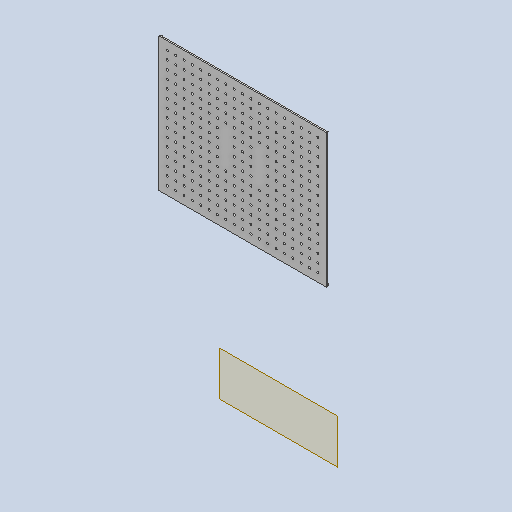
# Autodesk Inventor part: attachments_hub
Saved by Autodesk Inventor 2024.3 (Build 283343000, 343)
## iProperties
Created: 2026-05-03
Part Number: attachments_hub
Material: Generic
Document SubType Name: Modeling
Designer: owozn
Density: 1 g/cm^3
Appearance: Default
Author: owozn
Autodesk Inventor part; units mm, degrees
ref_plane "YZ Plane" through (0, 0, 0) normal (1, 0, 0) x (0, 1, 0)
ref_plane "XZ Plane" through (0, 0, 0) normal (0, 1, 0) x (-1, 0, 0)
ref_plane "XY Plane" through (0, 0, 0) normal (0, 0, 1) x (1, 0, 0)
ref_plane "Work Plane1" through (13.6818, -331.3189, 0) normal (0, 0, 1) x (1, 0, 0)
sketch "Sketch1" plane through (13.6818, -331.3189, 0) normal (0, 0, 1) x (1, 0, 0)
  line L0 (-13.6818, 214.2062) -> (-13.6818, 284.2062) projected
  line L1 (-49.9333, 331.3189) -> (45.2667, 331.3189) projected
  line L2 (-47.6818, 361.3189) -> (-37.6818, 361.3189)
  line L3 (-37.6818, 361.3189) -> (-37.6818, 311.3189)
  line L4 (-37.6818, 311.3189) -> (-47.6818, 311.3189)
  line L5 (-47.6818, 311.3189) -> (-47.6818, 361.3189)
  line L6 (-47.6818, 361.3189) -> (-37.6818, 311.3189) construction
  line L7 (-37.6818, 361.3189) -> (-47.6818, 311.3189) construction
  line L8 (20.3182, 361.3189) -> (10.3182, 361.3189)
  line L9 (10.3182, 361.3189) -> (10.3182, 311.3189)
  line L10 (10.3182, 311.3189) -> (20.3182, 311.3189)
  line L11 (20.3182, 311.3189) -> (20.3182, 361.3189)
  line L12 (20.3182, 361.3189) -> (10.3182, 311.3189) construction
  line L13 (10.3182, 361.3189) -> (20.3182, 311.3189) construction
  point P0 (-13.6818, 331.3189)
  point P1 (-42.6818, 336.3189)
  point P2 (15.3182, 336.3189)
  dimension "d0" = 10
  dimension "d1" = 50
  dimension "d2" = 29
  dimension "d3" = 5
  constraints: 24 end point, 5 symmetric about line, 2 midpoint, 2 parallel, 1 horizontal, 1 perpendicular
  measures "d0" distance of L3.end L4.end
  measures "d1" distance of L2.end L3.end
  measures "d2" distance from line of L0 point (-42.682, 336.319)
  measures "d3" distance from line of L1 point (-42.682, 336.319)
extrude "Extrusion1" add sketch "Sketch1" along normal blind 35
sketch "Sketch2" plane through (24, -20, 0) normal (-1, 0, 0) x (0, 0, 1)
  line L0 (0, -10) -> (0, 60) projected
  line L1 (-7, 20) -> (42, 20) projected
  circle A0 centre (7, 25) radius 1.6
  circle A1 centre (7, 41) radius 1.6
  line L2 (8.6, 25) -> (8.6, 41)
  line L3 (5.4, 25) -> (5.4, 41)
  point P0 (0, 20)
  dimension "d6" = 3.2
  dimension "d7" = 3.2
  dimension "d8" = 7
  dimension "d9" = 7
  dimension "d10" = 21
  dimension "d11" = 5
  constraints: 4 end point, 4 point on circle, 4 tangent, 2 centre point
  measures "d6" diameter of A0
  measures "d7" diameter of A1
  measures "d8" distance from line of L0 A0.centre
  measures "d9" distance from line of L0 A1.centre
  measures "d10" distance from line of L1 A1.centre
  measures "d11" distance from line of L1 A0.centre
extrude "Extrusion2" cut sketch "Sketch2" along normal through all both and the other way through all
sketch "Sketch3" plane through (13.6818, -331.3189, 35) normal (0, 0, 1) x (1, 0, 0)
  line L0 (-13.6818, 100.7837) -> (-13.6818, 404.7415) projected
  line L1 (-177.3333, 331.3189) -> (172.6667, 331.3189) projected
  line L2 (111.3182, 231.3189) -> (-138.6818, 231.3189)
  line L3 (-138.6818, 231.3189) -> (-138.6818, 431.3189)
  line L4 (-138.6818, 431.3189) -> (111.3182, 431.3189)
  line L5 (111.3182, 431.3189) -> (111.3182, 231.3189)
  line L6 (111.3182, 231.3189) -> (-138.6818, 431.3189) construction
  line L7 (-138.6818, 231.3189) -> (111.3182, 431.3189) construction
  circle A0 centre (-126.1818, 418.8189) radius 1.6
  circle A1 centre (-113.6818, 418.8189) radius 1.6
  circle A2 centre (-101.1818, 418.8189) radius 1.6
  circle A3 centre (-88.6818, 418.8189) radius 1.6
  circle A4 centre (-76.1818, 418.8189) radius 1.6
  circle A5 centre (-63.6818, 418.8189) radius 1.6
  circle A6 centre (-51.1818, 418.8189) radius 1.6
  circle A7 centre (-38.6818, 418.8189) radius 1.6
  circle A8 centre (-26.1818, 418.8189) radius 1.6
  circle A9 centre (-13.6818, 418.8189) radius 1.6
  circle A10 centre (-1.1818, 418.8189) radius 1.6
  circle A11 centre (11.3182, 418.8189) radius 1.6
  circle A12 centre (23.8182, 418.8189) radius 1.6
  circle A13 centre (36.3182, 418.8189) radius 1.6
  circle A14 centre (48.8182, 418.8189) radius 1.6
  circle A15 centre (61.3182, 418.8189) radius 1.6
  circle A16 centre (73.8182, 418.8189) radius 1.6
  circle A17 centre (86.3182, 418.8189) radius 1.6
  circle A18 centre (98.8182, 418.8189) radius 1.6
  circle A19 centre (-126.1818, 406.3189) radius 1.6
  circle A20 centre (-113.6818, 406.3189) radius 1.6
  circle A21 centre (-101.1818, 406.3189) radius 1.6
  circle A22 centre (-88.6818, 406.3189) radius 1.6
  circle A23 centre (-76.1818, 406.3189) radius 1.6
  circle A24 centre (-63.6818, 406.3189) radius 1.6
  circle A25 centre (-51.1818, 406.3189) radius 1.6
  circle A26 centre (-38.6818, 406.3189) radius 1.6
  circle A27 centre (-26.1818, 406.3189) radius 1.6
  circle A28 centre (-13.6818, 406.3189) radius 1.6
  circle A29 centre (-1.1818, 406.3189) radius 1.6
  circle A30 centre (11.3182, 406.3189) radius 1.6
  circle A31 centre (23.8182, 406.3189) radius 1.6
  circle A32 centre (36.3182, 406.3189) radius 1.6
  circle A33 centre (48.8182, 406.3189) radius 1.6
  circle A34 centre (61.3182, 406.3189) radius 1.6
  circle A35 centre (73.8182, 406.3189) radius 1.6
  circle A36 centre (86.3182, 406.3189) radius 1.6
  circle A37 centre (98.8182, 406.3189) radius 1.6
  circle A38 centre (-126.1818, 393.8189) radius 1.6
  circle A39 centre (-113.6818, 393.8189) radius 1.6
  circle A40 centre (-101.1818, 393.8189) radius 1.6
  circle A41 centre (-88.6818, 393.8189) radius 1.6
  circle A42 centre (-76.1818, 393.8189) radius 1.6
  circle A43 centre (-63.6818, 393.8189) radius 1.6
  circle A44 centre (-51.1818, 393.8189) radius 1.6
  circle A45 centre (-38.6818, 393.8189) radius 1.6
  circle A46 centre (-26.1818, 393.8189) radius 1.6
  circle A47 centre (-13.6818, 393.8189) radius 1.6
  circle A48 centre (-1.1818, 393.8189) radius 1.6
  circle A49 centre (11.3182, 393.8189) radius 1.6
  circle A50 centre (23.8182, 393.8189) radius 1.6
  circle A51 centre (36.3182, 393.8189) radius 1.6
  circle A52 centre (48.8182, 393.8189) radius 1.6
  circle A53 centre (61.3182, 393.8189) radius 1.6
  circle A54 centre (73.8182, 393.8189) radius 1.6
  circle A55 centre (86.3182, 393.8189) radius 1.6
  circle A56 centre (98.8182, 393.8189) radius 1.6
  circle A57 centre (-126.1818, 381.3189) radius 1.6
  circle A58 centre (-113.6818, 381.3189) radius 1.6
  circle A59 centre (-101.1818, 381.3189) radius 1.6
  circle A60 centre (-88.6818, 381.3189) radius 1.6
  circle A61 centre (-76.1818, 381.3189) radius 1.6
  circle A62 centre (-63.6818, 381.3189) radius 1.6
  circle A63 centre (-51.1818, 381.3189) radius 1.6
  circle A64 centre (-38.6818, 381.3189) radius 1.6
  circle A65 centre (-26.1818, 381.3189) radius 1.6
  circle A66 centre (-13.6818, 381.3189) radius 1.6
  circle A67 centre (-1.1818, 381.3189) radius 1.6
  circle A68 centre (11.3182, 381.3189) radius 1.6
  circle A69 centre (23.8182, 381.3189) radius 1.6
  circle A70 centre (36.3182, 381.3189) radius 1.6
  circle A71 centre (48.8182, 381.3189) radius 1.6
  circle A72 centre (61.3182, 381.3189) radius 1.6
  circle A73 centre (73.8182, 381.3189) radius 1.6
  circle A74 centre (86.3182, 381.3189) radius 1.6
  circle A75 centre (98.8182, 381.3189) radius 1.6
  circle A76 centre (-126.1818, 368.8189) radius 1.6
  circle A77 centre (-113.6818, 368.8189) radius 1.6
  circle A78 centre (-101.1818, 368.8189) radius 1.6
  circle A79 centre (-88.6818, 368.8189) radius 1.6
  circle A80 centre (-76.1818, 368.8189) radius 1.6
  circle A81 centre (-63.6818, 368.8189) radius 1.6
  circle A82 centre (-51.1818, 368.8189) radius 1.6
  circle A83 centre (-38.6818, 368.8189) radius 1.6
  circle A84 centre (-26.1818, 368.8189) radius 1.6
  circle A85 centre (-13.6818, 368.8189) radius 1.6
  circle A86 centre (-1.1818, 368.8189) radius 1.6
  circle A87 centre (11.3182, 368.8189) radius 1.6
  circle A88 centre (23.8182, 368.8189) radius 1.6
  circle A89 centre (36.3182, 368.8189) radius 1.6
  circle A90 centre (48.8182, 368.8189) radius 1.6
  circle A91 centre (61.3182, 368.8189) radius 1.6
  circle A92 centre (73.8182, 368.8189) radius 1.6
  circle A93 centre (86.3182, 368.8189) radius 1.6
  circle A94 centre (98.8182, 368.8189) radius 1.6
  circle A95 centre (-126.1818, 356.3189) radius 1.6
  circle A96 centre (-113.6818, 356.3189) radius 1.6
  circle A97 centre (-101.1818, 356.3189) radius 1.6
  circle A98 centre (-88.6818, 356.3189) radius 1.6
  circle A99 centre (-76.1818, 356.3189) radius 1.6
  circle A100 centre (-63.6818, 356.3189) radius 1.6
  circle A101 centre (-51.1818, 356.3189) radius 1.6
  circle A102 centre (-38.6818, 356.3189) radius 1.6
  circle A103 centre (-26.1818, 356.3189) radius 1.6
  circle A104 centre (-13.6818, 356.3189) radius 1.6
  circle A105 centre (-1.1818, 356.3189) radius 1.6
  circle A106 centre (11.3182, 356.3189) radius 1.6
  circle A107 centre (23.8182, 356.3189) radius 1.6
  circle A108 centre (36.3182, 356.3189) radius 1.6
  circle A109 centre (48.8182, 356.3189) radius 1.6
  circle A110 centre (61.3182, 356.3189) radius 1.6
  circle A111 centre (73.8182, 356.3189) radius 1.6
  circle A112 centre (86.3182, 356.3189) radius 1.6
  circle A113 centre (98.8182, 356.3189) radius 1.6
  circle A114 centre (-126.1818, 343.8189) radius 1.6
  circle A115 centre (-113.6818, 343.8189) radius 1.6
  circle A116 centre (-101.1818, 343.8189) radius 1.6
  circle A117 centre (-88.6818, 343.8189) radius 1.6
  circle A118 centre (-76.1818, 343.8189) radius 1.6
  circle A119 centre (-63.6818, 343.8189) radius 1.6
  circle A120 centre (-51.1818, 343.8189) radius 1.6
  circle A121 centre (-38.6818, 343.8189) radius 1.6
  circle A122 centre (-26.1818, 343.8189) radius 1.6
  circle A123 centre (-13.6818, 343.8189) radius 1.6
  circle A124 centre (-1.1818, 343.8189) radius 1.6
  circle A125 centre (11.3182, 343.8189) radius 1.6
  circle A126 centre (23.8182, 343.8189) radius 1.6
  circle A127 centre (36.3182, 343.8189) radius 1.6
  circle A128 centre (48.8182, 343.8189) radius 1.6
  circle A129 centre (61.3182, 343.8189) radius 1.6
  circle A130 centre (73.8182, 343.8189) radius 1.6
  circle A131 centre (86.3182, 343.8189) radius 1.6
  circle A132 centre (98.8182, 343.8189) radius 1.6
  circle A133 centre (-126.1818, 331.3189) radius 1.6
  circle A134 centre (-113.6818, 331.3189) radius 1.6
  circle A135 centre (-101.1818, 331.3189) radius 1.6
  circle A136 centre (-88.6818, 331.3189) radius 1.6
  circle A137 centre (-76.1818, 331.3189) radius 1.6
  circle A138 centre (-63.6818, 331.3189) radius 1.6
  circle A139 centre (-51.1818, 331.3189) radius 1.6
  circle A140 centre (-38.6818, 331.3189) radius 1.6
  circle A141 centre (-26.1818, 331.3189) radius 1.6
  circle A142 centre (-13.6818, 331.3189) radius 1.6
  circle A143 centre (-1.1818, 331.3189) radius 1.6
  circle A144 centre (11.3182, 331.3189) radius 1.6
  circle A145 centre (23.8182, 331.3189) radius 1.6
  circle A146 centre (36.3182, 331.3189) radius 1.6
  circle A147 centre (48.8182, 331.3189) radius 1.6
  circle A148 centre (61.3182, 331.3189) radius 1.6
  circle A149 centre (73.8182, 331.3189) radius 1.6
  circle A150 centre (86.3182, 331.3189) radius 1.6
  circle A151 centre (98.8182, 331.3189) radius 1.6
  circle A152 centre (-126.1818, 318.8189) radius 1.6
  circle A153 centre (-113.6818, 318.8189) radius 1.6
  circle A154 centre (-101.1818, 318.8189) radius 1.6
  circle A155 centre (-88.6818, 318.8189) radius 1.6
  circle A156 centre (-76.1818, 318.8189) radius 1.6
  circle A157 centre (-63.6818, 318.8189) radius 1.6
  circle A158 centre (-51.1818, 318.8189) radius 1.6
  circle A159 centre (-38.6818, 318.8189) radius 1.6
  circle A160 centre (-26.1818, 318.8189) radius 1.6
  circle A161 centre (-13.6818, 318.8189) radius 1.6
  circle A162 centre (-1.1818, 318.8189) radius 1.6
  circle A163 centre (11.3182, 318.8189) radius 1.6
  circle A164 centre (23.8182, 318.8189) radius 1.6
  circle A165 centre (36.3182, 318.8189) radius 1.6
  circle A166 centre (48.8182, 318.8189) radius 1.6
  circle A167 centre (61.3182, 318.8189) radius 1.6
  circle A168 centre (73.8182, 318.8189) radius 1.6
  circle A169 centre (86.3182, 318.8189) radius 1.6
  circle A170 centre (98.8182, 318.8189) radius 1.6
  circle A171 centre (-126.1818, 306.3189) radius 1.6
  circle A172 centre (-113.6818, 306.3189) radius 1.6
  circle A173 centre (-101.1818, 306.3189) radius 1.6
  circle A174 centre (-88.6818, 306.3189) radius 1.6
  circle A175 centre (-76.1818, 306.3189) radius 1.6
  circle A176 centre (-63.6818, 306.3189) radius 1.6
  circle A177 centre (-51.1818, 306.3189) radius 1.6
  circle A178 centre (-38.6818, 306.3189) radius 1.6
  circle A179 centre (-26.1818, 306.3189) radius 1.6
  circle A180 centre (-13.6818, 306.3189) radius 1.6
  circle A181 centre (-1.1818, 306.3189) radius 1.6
  circle A182 centre (11.3182, 306.3189) radius 1.6
  circle A183 centre (23.8182, 306.3189) radius 1.6
  circle A184 centre (36.3182, 306.3189) radius 1.6
  circle A185 centre (48.8182, 306.3189) radius 1.6
  circle A186 centre (61.3182, 306.3189) radius 1.6
  circle A187 centre (73.8182, 306.3189) radius 1.6
  circle A188 centre (86.3182, 306.3189) radius 1.6
  circle A189 centre (98.8182, 306.3189) radius 1.6
  circle A190 centre (-126.1818, 293.8189) radius 1.6
  circle A191 centre (-113.6818, 293.8189) radius 1.6
  circle A192 centre (-101.1818, 293.8189) radius 1.6
  circle A193 centre (-88.6818, 293.8189) radius 1.6
  circle A194 centre (-76.1818, 293.8189) radius 1.6
  circle A195 centre (-63.6818, 293.8189) radius 1.6
  circle A196 centre (-51.1818, 293.8189) radius 1.6
  circle A197 centre (-38.6818, 293.8189) radius 1.6
  circle A198 centre (-26.1818, 293.8189) radius 1.6
  circle A199 centre (-13.6818, 293.8189) radius 1.6
  circle A200 centre (-1.1818, 293.8189) radius 1.6
  circle A201 centre (11.3182, 293.8189) radius 1.6
  circle A202 centre (23.8182, 293.8189) radius 1.6
  circle A203 centre (36.3182, 293.8189) radius 1.6
  circle A204 centre (48.8182, 293.8189) radius 1.6
  circle A205 centre (61.3182, 293.8189) radius 1.6
  circle A206 centre (73.8182, 293.8189) radius 1.6
  circle A207 centre (86.3182, 293.8189) radius 1.6
  circle A208 centre (98.8182, 293.8189) radius 1.6
  circle A209 centre (-126.1818, 281.3189) radius 1.6
  circle A210 centre (-113.6818, 281.3189) radius 1.6
  circle A211 centre (-101.1818, 281.3189) radius 1.6
  circle A212 centre (-88.6818, 281.3189) radius 1.6
  circle A213 centre (-76.1818, 281.3189) radius 1.6
  circle A214 centre (-63.6818, 281.3189) radius 1.6
  circle A215 centre (-51.1818, 281.3189) radius 1.6
  circle A216 centre (-38.6818, 281.3189) radius 1.6
  circle A217 centre (-26.1818, 281.3189) radius 1.6
  circle A218 centre (-13.6818, 281.3189) radius 1.6
  circle A219 centre (-1.1818, 281.3189) radius 1.6
  circle A220 centre (11.3182, 281.3189) radius 1.6
  circle A221 centre (23.8182, 281.3189) radius 1.6
  circle A222 centre (36.3182, 281.3189) radius 1.6
  circle A223 centre (48.8182, 281.3189) radius 1.6
  circle A224 centre (61.3182, 281.3189) radius 1.6
  circle A225 centre (73.8182, 281.3189) radius 1.6
  circle A226 centre (86.3182, 281.3189) radius 1.6
  circle A227 centre (98.8182, 281.3189) radius 1.6
  circle A228 centre (-126.1818, 268.8189) radius 1.6
  circle A229 centre (-113.6818, 268.8189) radius 1.6
  circle A230 centre (-101.1818, 268.8189) radius 1.6
  circle A231 centre (-88.6818, 268.8189) radius 1.6
  circle A232 centre (-76.1818, 268.8189) radius 1.6
  circle A233 centre (-63.6818, 268.8189) radius 1.6
  circle A234 centre (-51.1818, 268.8189) radius 1.6
  circle A235 centre (-38.6818, 268.8189) radius 1.6
  circle A236 centre (-26.1818, 268.8189) radius 1.6
  circle A237 centre (-13.6818, 268.8189) radius 1.6
  circle A238 centre (-1.1818, 268.8189) radius 1.6
  circle A239 centre (11.3182, 268.8189) radius 1.6
  circle A240 centre (23.8182, 268.8189) radius 1.6
  circle A241 centre (36.3182, 268.8189) radius 1.6
  circle A242 centre (48.8182, 268.8189) radius 1.6
  circle A243 centre (61.3182, 268.8189) radius 1.6
  circle A244 centre (73.8182, 268.8189) radius 1.6
  circle A245 centre (86.3182, 268.8189) radius 1.6
  circle A246 centre (98.8182, 268.8189) radius 1.6
  circle A247 centre (-126.1818, 256.3189) radius 1.6
  circle A248 centre (-113.6818, 256.3189) radius 1.6
  circle A249 centre (-101.1818, 256.3189) radius 1.6
  circle A250 centre (-88.6818, 256.3189) radius 1.6
  circle A251 centre (-76.1818, 256.3189) radius 1.6
  circle A252 centre (-63.6818, 256.3189) radius 1.6
  circle A253 centre (-51.1818, 256.3189) radius 1.6
  circle A254 centre (-38.6818, 256.3189) radius 1.6
  circle A255 centre (-26.1818, 256.3189) radius 1.6
  circle A256 centre (-13.6818, 256.3189) radius 1.6
  circle A257 centre (-1.1818, 256.3189) radius 1.6
  circle A258 centre (11.3182, 256.3189) radius 1.6
  circle A259 centre (23.8182, 256.3189) radius 1.6
  circle A260 centre (36.3182, 256.3189) radius 1.6
  circle A261 centre (48.8182, 256.3189) radius 1.6
  circle A262 centre (61.3182, 256.3189) radius 1.6
  circle A263 centre (73.8182, 256.3189) radius 1.6
  circle A264 centre (86.3182, 256.3189) radius 1.6
  circle A265 centre (98.8182, 256.3189) radius 1.6
  circle A266 centre (-126.1818, 243.8189) radius 1.6
  circle A267 centre (-113.6818, 243.8189) radius 1.6
  circle A268 centre (-101.1818, 243.8189) radius 1.6
  circle A269 centre (-88.6818, 243.8189) radius 1.6
  circle A270 centre (-76.1818, 243.8189) radius 1.6
  circle A271 centre (-63.6818, 243.8189) radius 1.6
  circle A272 centre (-51.1818, 243.8189) radius 1.6
  circle A273 centre (-38.6818, 243.8189) radius 1.6
  circle A274 centre (-26.1818, 243.8189) radius 1.6
  circle A275 centre (-13.6818, 243.8189) radius 1.6
  circle A276 centre (-1.1818, 243.8189) radius 1.6
  circle A277 centre (11.3182, 243.8189) radius 1.6
  circle A278 centre (23.8182, 243.8189) radius 1.6
  circle A279 centre (36.3182, 243.8189) radius 1.6
  circle A280 centre (48.8182, 243.8189) radius 1.6
  circle A281 centre (61.3182, 243.8189) radius 1.6
  circle A282 centre (73.8182, 243.8189) radius 1.6
  circle A283 centre (86.3182, 243.8189) radius 1.6
  circle A284 centre (98.8182, 243.8189) radius 1.6
  point P0 (-13.6818, 331.3189)
  dimension "d14" = 250
  dimension "d15" = 200
  dimension "d19" = 3.2
  dimension "d20" = 12.5
  dimension "d21" = 12.5
  dimension "d24" = 12.5
  dimension "d27" = 12.5
  constraints: 285 centre point, 12 end point, 2 horizontal, 2 midpoint, 2 parallel, 1 perpendicular, 1 vertical, 568 other
  measures "d14" distance of L3.end L4.end
  measures "d15" distance of L2.end L3.end
  measures "d19" diameter of A0
  measures "d20" distance from line of L4 A0.centre
  measures "d21" distance from line of L3 A0.centre
  measures "d24" distance of A0.centre A1.centre
  measures "d27" distance of A0.centre A19.centre
extrude "Extrusion3" add sketch "Sketch3" along normal blind 5 contours L2 L3 L1 A133 A134 A135 A136 A137 A138 A139 A140 A141 A142 L0 A161 A180 A199 A218 A237 A256 A275 | L0 A275 A256 A237 A218 A199 A180 A161 A142 L1 A143 A144 A145 A146 A147 A148 A149 A150 A151 L5 L2 | L1 A151 A150 A149 A148 A147 A146 A145 A144 A143 A142 A141 A140 A139 A138 A137 A136 A135 A134 A133 L3 L4 L5 | A144 L1 | L1 A144 | A140 L1 | L1 A140 | A102 | A106 | A121 | A125 | A159 | A163
fillet "Fillet2" radius 3 12 edges at (-24, -20, 17.5) (-34, -20, 17.5) (-34, 30, 17.5) (-24, 30, 17.5) (24, -20, 17.5) (24, 30, 17.5) (34, 30, 17.5) (34, -20, 17.5) (0, -100, 35) (125, 0, 35) (0, 100, 35) (-125, 0, 35)
fillet "Fillet3" radius 2 16 edges at (-24.8787, 29.1213, 35) (-29, 30, 35) (-33.1213, 29.1213, 35) (-34, 5, 35) (-33.1213, -19.1213, 35) (-29, -20, 35) (-24.8787, -19.1213, 35) (-24, 5, 35) (34, 5, 35) (33.1213, -19.1213, 35) (29, -20, 35) (24.8787, -19.1213, 35) (24, 5, 35) (24.8787, 29.1213, 35) (29, 30, 35) (33.1213, 29.1213, 35)
body "Solid1"
